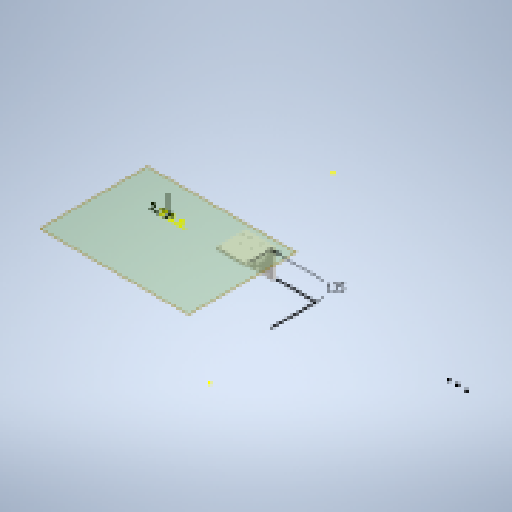
# Autodesk Inventor part: крепление свободной шестерни
Saved by Autodesk Inventor 2024.2 (Build 282272000, 272)
## iProperties
Created: 2025-11-23
Part Number: крепление свободной шестерни
Material: Типовые
Document SubType Name: Modeling
Designer: katya_notebook
Density: 1 g/cm^3
Appearance: По умолчанию
Mass: 30.8314 g
Surface Area: 144.895 cm^2
Volume: 30.8314 cm^3
Author: katya_notebook
Autodesk Inventor part; units mm, degrees
ref_plane "YZ Plane" through (0, 0, 0) normal (1, 0, 0) x (0, 1, 0)
ref_plane "XZ Plane" through (0, 0, 0) normal (0, 1, 0) x (-1, 0, 0)
ref_plane "XY Plane" through (0, 0, 0) normal (0, 0, 1) x (1, 0, 0)
ref_plane "РабПлоскость1" through (-232.05, -185.1645, -149.0585) normal (0, -1, 0) x (1, 0, 0)
sketch "Эскиз1" plane through (-232.05, -185.1645, -149.0585) normal (0, -1, 0) x (1, 0, 0)
  line L0 (-135, 97.5) -> (-135, 77.5) projected
  line L1 (-118.5237, -91) -> (-118.5237, -37.5) projected
  line L2 (-135, -79.6587) -> (-135, -55.4979)
  line L3 (-118.5237, -55.4979) -> (-118.5237, -79.6587)
  line L4 (-118.5237, -55.4979) -> (-135, -55.4979)
  line L5 (-0.1223, -79.6587) -> (-0.1223, 72.5986)
  line L6 (118.2792, -55.4979) -> (134.7555, -55.4979)
  line L7 (-118.5237, -97.5) -> (-58.5237, -97.5) projected
  line L8 (118.2792, -97.5) -> (58.2792, -97.5)
  line L9 (58.2792, -97.5) -> (58.2792, -37.5)
  line L10 (58.2792, -37.5) -> (118.2792, -37.5)
  line L11 (118.2792, -37.5) -> (118.2792, -97.5)
  point P0 (232.05, 149.0585)
  point P1 (118.2792, -37.5)
  dimension "d5" = 135
  dimension "d13" = 135
  dimension "d1" = 60
  dimension "d2" = 60
  constraints: 18 end point, 4 point on line, 3 symmetric about line, 2 parallel, 2 perpendicular, 1 horizontal, 1 vertical
  measures "d1" distance of L10.end L8.start
  measures "d2" distance of L9.end L10.end
ref_plane "РабПлоскость2" through (-334.9307, -190.1645, -233.6585) normal (0, 1, 0) x (0, 0, 1)
extrude "Выдавливание1" add sketch "Эскиз1" along normal up to surface (5 mm away)
sketch "Эскиз2" plane through (-173.7708, -190.1645, -186.5585) normal (0, -1, 0) x (1, 0, 0)
  circle A0 centre (-172.803, -47.5) radius 2 projected
  circle A1 centre (-120.803, -47.5) radius 2 projected
  circle A2 centre (-120.803, -5) radius 2 projected
  circle A3 centre (-172.803, -5) radius 2 projected
  line L0 (-193.2792, 135) -> (-193.2792, 115) projected
  line L1 (76.7208, -52) -> (76.7208, 127) projected
  line L2 (-193.2792, 115) -> (-58.2792, 115)
  line L3 (-58.2792, 115) -> (-58.2792, 207.9889)
  circle A4 centre (56.2445, -47.5) radius 2
  circle A5 centre (4.2445, -47.5) radius 2
  circle A6 centre (4.2445, -5) radius 2
  circle A7 centre (56.2445, -5) radius 2
  point P0 (173.7708, 186.5585)
  dimension "d5" = 135
  constraints: 4 centre point, 4 end point, 4 symmetric about line, 1 horizontal, 1 vertical, 4 other
  measures "d5" distance of L0.end L2.end
extrude "Выдавливание2" cut sketch "Эскиз2" against normal blind 10 contours A4 | A5 | A6 | A7
sketch "Эскиз3" plane through (-173.7708, -190.1645, -186.5585) normal (0, -1, 0) x (1, 0, 0)
  line L0 (0, -60) -> (60, -60) projected
  line L1 (0, -60) -> (60, -60)
  line L2 (60, -60) -> (60, -53.5)
  line L3 (60, -53.5) -> (0, -53.5)
  line L4 (0, -53.5) -> (0, -60)
  point P0 (173.7708, 186.5585)
  dimension "d8" = 6.5
  constraints: 8 end point, 2 parallel, 1 horizontal, 1 perpendicular
  measures "d8" distance of L1.end L2.end
sketch "Эскиз4" plane through (-173.7708, -190.1645, -186.5585) normal (0, -1, 0) x (1, 0, 0)
  spline S0 degree 3 poles (43.2445, -30) (43.2445, -30.1203) (43.2336, -30.2387) (43.1929, -30.4661) (43.1631, -30.5751) (43.0528, -30.8816) (42.9505, -31.0587) (42.5833, -31.5484) (42.2402, -31.7817) (41.4641, -32.0292) (41.03, -32.0367) (40.4334, -31.8378) (40.2391, -31.7434) (39.8778, -31.4773) (39.7111, -31.305) (39.4834, -30.9643) (39.3942, -30.7855) (39.2746, -30.4002) (39.2445, -30.1935) (39.2445, -29.8065) (39.2746, -29.5998) (39.3942, -29.2145) (39.4834, -29.0357) (39.7111, -28.695) (39.8778, -28.5227) (40.2391, -28.2566) (40.4334, -28.1622) (41.03, -27.9633) (41.4641, -27.9708) (42.2402, -28.2183) (42.5833, -28.4516) (42.9505, -28.9413) (43.0528, -29.1184) (43.1631, -29.4249) (43.1929, -29.5339) (43.2336, -29.7613) (43.2445, -29.8797) (43.2445, -30) knots 0 0 0 0 0.036086 0.036086 0.072173 0.072173 0.144346 0.144346 0.322747 0.322747 0.501149 0.501149 0.577509 0.577509 0.653869 0.653869 0.711915 0.711915 0.769961 0.769961 0.828007 0.828007 0.886052 0.886052 0.962412 0.962412 1.038772 1.038772 1.217174 1.217174 1.395575 1.395575 1.467748 1.467748 1.503835 1.503835 1.539921 1.539921 1.539921 1.539921 projected
  spline S1 degree 3 poles (20.7277, -30) (20.7277, -30.1752) (20.703, -30.3631) (20.604, -30.7163) (20.53, -30.8816) (20.3402, -31.202) (20.1997, -31.3694) (19.8919, -31.6391) (19.7251, -31.7419) (19.1904, -31.9904) (18.7862, -32.034) (18.0457, -31.9171) (17.7092, -31.7574) (17.2213, -31.3457) (16.9969, -31.0683) (16.8255, -30.6264) (16.7899, -30.5111) (16.7409, -30.2621) (16.7277, -30.1279) (16.7277, -29.8721) (16.7409, -29.7379) (16.7899, -29.4889) (16.8255, -29.3736) (16.9969, -28.9317) (17.2213, -28.6543) (17.7092, -28.2426) (18.0457, -28.0829) (18.7862, -27.966) (19.1904, -28.0096) (19.7251, -28.2581) (19.8919, -28.3609) (20.1997, -28.6306) (20.3402, -28.798) (20.53, -29.1184) (20.604, -29.2837) (20.703, -29.6369) (20.7277, -29.8248) (20.7277, -30) knots 0 0 0 0 0.052568 0.052568 0.105137 0.105137 0.174601 0.174601 0.244066 0.244066 0.414781 0.414781 0.585496 0.585496 0.721852 0.721852 0.760221 0.760221 0.798591 0.798591 0.83696 0.83696 0.875329 0.875329 1.011685 1.011685 1.1824 1.1824 1.353115 1.353115 1.42258 1.42258 1.492044 1.492044 1.544613 1.544613 1.597181 1.597181 1.597181 1.597181 projected
  point P0 (173.7708, 186.5585)
  point P1 (43.2445, -30)
  point P2 (20.7277, -30)
extrude "Выдавливание3" cut sketch "Эскиз4" against normal blind 10
ref_plane "РабПлоскость3" through (-350.5737, -240.8695, -246.5585) normal (0, -1, 0) x (1, 0, 0)
extrude "Выдавливание4" add sketch "Эскиз3" along normal up to surface (50.705 mm away)
sketch "Эскиз5" plane through (-173.7708, -240.8695, -246.5585) normal (0, -1, 0) x (1, 0, 0)
  circle A0 centre (-164.803, 3.25) radius 1.75 projected
  circle A1 centre (-146.803, 3.25) radius 1.75 projected
  circle A2 centre (-128.803, 3.25) radius 1.75 projected
  line L0 (76.7208, 0) -> (4, 0) projected
  line L1 (4, 0) -> (139, 0)
  line L2 (139, 0) -> (139, 88.2878)
  circle A3 centre (442.803, 3.25) radius 1.75
  circle A4 centre (424.803, 3.25) radius 1.75
  circle A5 centre (406.803, 3.25) radius 1.75
  point P0 (173.7708, 246.5585)
  dimension "d13" = 135
  constraints: 4 end point, 3 centre point, 3 symmetric about line, 1 point on line, 1 vertical, 3 other
  measures "d13" distance of L1.end L0.end
ref_plane "РабПлоскость4" through (-340.3237, -230.8695, -245.0585) normal (0, -1, 0) x (1, 0, 0)
sketch "Эскиз6" plane through (-173.7708, -190.1645, -240.0585) normal (0, 0, 1) x (1, 0, 0)
  circle A0 centre (30.2445, -21) radius 2.5 projected
  circle A1 centre (30.2445, -21) radius 17.5
  point P0 (173.7708, 190.1645)
  dimension "d16" = 35
  constraints: 1 centre point, 1 coincident
  measures "d16" diameter of A1
extrude "Выдавливание6" cut sketch "Эскиз6" against normal blind 10 contours A0 | A1
sketch "Эскиз7" plane through (-113.7708, -185.1645, -246.5585) normal (0, 0, -1) x (-1, 0, 0)
  line L0 (228.053, -47.9768) -> (228.053, -50.9768) projected
  line L1 (228.053, -50.9768) -> (221.553, -50.9768) projected
  line L2 (221.553, -47.9768) -> (228.053, -47.9768) projected
  line L3 (221.553, -50.9768) -> (221.553, -47.9768) projected
  line L4 (210.053, -47.9768) -> (210.053, -50.9768) projected
  line L5 (210.053, -50.9768) -> (203.553, -50.9768) projected
  line L6 (203.553, -50.9768) -> (203.553, -47.9768) projected
  line L7 (203.553, -47.9768) -> (210.053, -47.9768) projected
  line L8 (192.053, -50.9768) -> (185.553, -50.9768) projected
  line L9 (185.553, -50.9768) -> (185.553, -47.9768) projected
  line L10 (185.553, -47.9768) -> (192.053, -47.9768) projected
  line L11 (192.053, -47.9768) -> (192.053, -50.9768) projected
  line L12 (253.2792, -59.705) -> (180.803, -59.705) projected
  line L13 (253.2792, -59.705) -> (217.0411, -59.705)
  line L14 (217.0411, -59.705) -> (217.0411, -16.367)
  line L15 (206.0292, -47.9768) -> (206.0292, -50.9768)
  line L16 (206.0292, -50.9768) -> (212.5292, -50.9768)
  line L17 (212.5292, -47.9768) -> (206.0292, -47.9768)
  line L18 (212.5292, -50.9768) -> (212.5292, -47.9768)
  line L19 (224.0292, -47.9768) -> (224.0292, -50.9768)
  line L20 (224.0292, -50.9768) -> (230.5292, -50.9768)
  line L21 (230.5292, -50.9768) -> (230.5292, -47.9768)
  line L22 (230.5292, -47.9768) -> (224.0292, -47.9768)
  line L23 (242.0292, -50.9768) -> (248.5292, -50.9768)
  line L24 (248.5292, -50.9768) -> (248.5292, -47.9768)
  line L25 (248.5292, -47.9768) -> (242.0292, -47.9768)
  line L26 (242.0292, -47.9768) -> (242.0292, -50.9768)
  point P0 (-113.7708, 185.1645)
  constraints: 28 end point, 12 symmetric about line, 1 midpoint, 1 vertical
sketch "Эскиз8" plane through (-173.7708, -240.8695, -240.0585) normal (0, 0, 1) x (1, 0, 0)
  circle A0 centre (30.2445, 29.705) radius 17.5 projected
  circle A1 centre (30.2445, 29.705) radius 7 projected
  point P0 (173.7708, 240.8695)
extrude "Выдавливание8" add sketch "Эскиз8" against normal up to surface (6.5 mm away)
sketch "Эскиз9" plane through (-173.7708, -240.8695, -240.0585) normal (0, 0, 1) x (1, 0, 0)
  arc A0 (37.3445, 29.705) -> (23.1445, 29.705) centre (30.2445, 29.705) ccw projected
  line L0 (37.3445, 29.705) -> (45.2445, 29.705) projected
  line L1 (45.2445, 29.705) -> (45.2445, 47.705) projected
  line L2 (45.2445, 47.705) -> (47.2445, 47.705) projected
  line L3 (50.2445, 50.705) -> (10.2445, 50.705) projected
  line L4 (13.2445, 47.705) -> (15.2445, 47.705) projected
  line L5 (15.2445, 47.705) -> (15.2445, 29.705) projected
  line L6 (15.2445, 29.705) -> (23.1445, 29.705) projected
  line L7 (50.2445, 50.705) -> (10.2445, 50.705) projected
  line L8 (45.2445, 47.705) -> (47.2445, 47.705) projected
  line L9 (13.2445, 47.705) -> (10.2445, 50.705) projected
  line L10 (50.2445, 50.705) -> (47.2445, 47.705) projected
  point P0 (173.7708, 240.8695)
ref_plane "РабПлоскость5" through (-163.5263, -211.1645, -221.5585) normal (0, 0, -1) x (0, 1, 0)
extrude "Выдавливание9" add sketch "Эскиз9" along normal up to surface (18.5 mm away)
sketch "Эскиз10" plane through (-136.4263, -211.1645, -240.0585) normal (0, -1, 0) x (1, 0, 0)
  spline S0 degree 3 poles (1.8953, 4.9991) (1.8944, 4.9137) (1.8996, 4.7356) (2.0298, 4.2824) (2.1169, 4.0707) (2.4403, 3.5783) (2.6648, 3.4214) (2.9132, 3.2437) (3.1329, 3.1315) (3.5962, 3.0266) (3.8627, 2.9863) (4.1292, 3.0061) (4.4485, 3.0497) (5.0812, 3.3629) (5.2298, 3.4915) (5.5261, 3.7869) (5.6407, 3.9862) (5.8212, 4.4108) (5.8776, 4.6475) (5.9089, 4.9522) (5.9108, 5.237) (5.6799, 5.9994) (5.5185, 6.1822) (5.3603, 6.3736) (5.2248, 6.5156) (4.7267, 6.8735) (4.3507, 6.9438) (3.9904, 7.0274) (3.8261, 7.0164) (3.4517, 6.9525) (3.1747, 6.8695) (2.784, 6.6748) (2.5802, 6.5307) (2.1778, 6.0657) (2.0816, 5.861) (1.9561, 5.4773) (1.8978, 5.2197) (1.8953, 4.9991) knots -0.617581 -0.617581 -0.617581 -0.617581 -0.591947 -0.591947 -0.573073 -0.573073 -0.540222 -0.540222 -0.491682 -0.491682 -0.466072 -0.466072 -0.460987 -0.460987 -0.456841 -0.456841 -0.449459 -0.449459 -0.440712 -0.440712 -0.435051 -0.435051 -0.427631 -0.427631 -0.418066 -0.418066 -0.393854 -0.393854 -0.318016 -0.318016 -0.225773 -0.225773 -0.149383 -0.149383 -0.066183 -0.066183 0 0 0 0 projected
  spline S1 degree 3 poles (-20.1358, 3.7018) (-19.9784, 3.5244) (-19.7373, 3.3185) (-19.2566, 3.083) (-19.0243, 3.0322) (-18.5989, 2.9904) (-18.3448, 2.9908) (-17.7198, 3.1844) (-17.5007, 3.3292) (-17.0322, 3.7216) (-16.879, 4.0055) (-16.7767, 4.2042) (-16.6834, 4.4333) (-16.6099, 4.8657) (-16.5909, 5.1119) (-16.7143, 5.6401) (-16.8009, 5.9009) (-17.121, 6.3482) (-17.3048, 6.5302) (-17.7894, 6.8514) (-18.0589, 6.9288) (-18.5717, 7.027) (-18.8341, 6.997) (-19.1764, 6.9243) (-19.3925, 6.8581) (-19.6812, 6.7033) (-19.8978, 6.5777) (-20.2684, 6.122) (-20.4032, 5.9367) (-20.5197, 5.6478) (-20.6106, 5.4165) (-20.6111, 4.6497) (-20.535, 4.4029) (-20.3432, 3.9448) (-20.1819, 3.7538) (-20.1358, 3.7018) knots -1.840358 -1.840358 -1.840358 -1.840358 -1.769222 -1.769222 -1.709875 -1.709875 -1.656566 -1.656566 -1.604902 -1.604902 -1.500987 -1.500987 -1.176684 -1.176684 -0.960047 -0.960047 -0.825926 -0.825926 -0.728108 -0.728108 -0.603604 -0.603604 -0.389887 -0.389887 -0.189621 -0.189621 -0.087541 -0.087541 -0.045854 -0.045854 -0.032602 -0.032602 -0.020855 -0.020855 0 0 0 0 projected
  point P0 (136.4263, 240.0585)
  point P1 (1.8953, 4.9991)
  point P2 (-20.1358, 3.7018)
extrude "Выдавливание10" cut sketch "Эскиз10" against normal up to surface (26 mm away)
sketch "Эскиз11" plane through (-113.7708, -185.1645, -246.5585) normal (0, 0, -1) x (-1, 0, 0)
  line L0 (228.053, -47.9768) -> (228.053, -50.9768) projected
  line L1 (228.053, -50.9768) -> (221.553, -50.9768) projected
  line L2 (221.553, -47.9768) -> (228.053, -47.9768) projected
  line L3 (221.553, -50.9768) -> (221.553, -47.9768) projected
  line L4 (210.053, -47.9768) -> (210.053, -50.9768) projected
  line L5 (210.053, -50.9768) -> (203.553, -50.9768) projected
  line L6 (203.553, -50.9768) -> (203.553, -47.9768) projected
  circle A0 centre (206.8029, -26) radius 22 construction
  line L7 (203.553, -47.9768) -> (210.053, -47.9768) projected
  line L8 (192.053, -47.9768) -> (192.053, -50.9768) projected
  line L9 (192.053, -50.9768) -> (185.553, -50.9768) projected
  line L10 (185.553, -47.9768) -> (192.053, -47.9768) projected
  line L11 (185.553, -50.9768) -> (185.553, -47.9768) projected
  line L12 (118.2792, -176.2779) -> (118.2792, 75.7221)
  line L13 (8.5055, -47.9768) -> (8.5055, -50.9768)
  line L14 (8.5055, -50.9768) -> (15.0055, -50.9768)
  line L15 (15.0055, -47.9768) -> (8.5055, -47.9768)
  line L16 (15.0055, -50.9768) -> (15.0055, -47.9768)
  line L17 (26.5055, -47.9768) -> (26.5055, -50.9768)
  line L18 (26.5055, -50.9768) -> (33.0055, -50.9768)
  line L19 (33.0055, -50.9768) -> (33.0055, -47.9768)
  line L20 (33.0055, -47.9768) -> (26.5055, -47.9768)
  line L21 (44.5055, -47.9768) -> (44.5055, -50.9768)
  line L22 (44.5055, -50.9768) -> (51.0055, -50.9768)
  line L23 (51.0055, -47.9768) -> (44.5055, -47.9768)
  line L24 (51.0055, -50.9768) -> (51.0055, -47.9768)
  point P0 (-113.7708, 185.1645)
  constraints: 26 end point, 12 symmetric about line, 1 vertical, 2 other
extrude "Выдавливание11" cut sketch "Эскиз11" against normal blind 10 contours L15 L16 L14 L13 | L20 L19 L18 L17 | L23 L24 L22 L21
sketch "Эскиз12" plane through (-173.7708, -240.8695, -246.5585) normal (0, -1, 0) x (1, 0, 0)
  circle A0 centre (48.2445, 3.25) radius 1.75
  circle A1 centre (30.2445, 3.25) radius 1.75
  circle A2 centre (12.2445, 3.25) radius 1.75
  point P0 (173.7708, 246.5585)
  constraints: 3 centre point
extrude "Выдавливание12" cut sketch "Эскиз12" against normal blind 10
